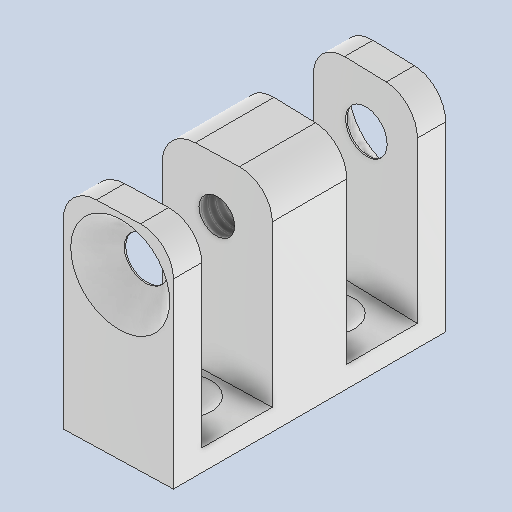
# Autodesk Inventor part: HalterUmlenkrolleDPL
Saved by Autodesk Inventor 2025 (Build 290162010, 162A)
## iProperties
Created: 2024-11-18
Part Number: HalterUmlenkrolleDPL
Material: PC/ABS-Kunststoff, 3DDruck, PLA
Document SubType Name: Modeling
Designer: Admin
Density: 1.1 g/cm^3
Appearance: Glatt - Weiß(2)
Mass: 2.69194 g
Surface Area: 21.9285 cm^2
Volume: 2.44721 cm^3
Author: Admin
Autodesk Inventor part; units mm, degrees
ref_plane "YZ Plane" through (0, 0, 0) normal (1, 0, 0) x (0, 1, 0)
ref_plane "XZ Plane" through (0, 0, 0) normal (0, 1, 0) x (-1, 0, 0)
ref_plane "XY Plane" through (0, 0, 0) normal (0, 0, 1) x (1, 0, 0)
sketch "Skizze1" plane through (0, 0, 0) normal (0, 0, 1) x (1, 0, 0)
  line L0 (12.8939, 29.9395) -> (2.8939, 30.2214)
  line L1 (2.8939, 30.2214) -> (2.8939, 27.5839)
  line L2 (2.8939, 27.5839) -> (12.8939, 27.302)
  line L3 (12.8939, 27.302) -> (12.8939, 29.9395)
  line L4 (12.8939, 7.1408) -> (2.8939, 6.8589)
  line L5 (2.8939, 6.8589) -> (2.8939, 4.2214)
  line L6 (2.8939, 4.2214) -> (12.8939, 4.5032)
  line L7 (12.8939, 4.5032) -> (12.8939, 7.1408)
  line L8 (2.8939, 20.9812) -> (12.8939, 20.6994)
  line L9 (12.8939, 13.7434) -> (2.8939, 13.4615)
  line L10 (16.8903, 10.5547) -> (7.8939, 10.3011) construction
  line L11 (16.8903, 23.888) -> (7.8939, 24.1416) construction
  line L12 (16.8903, 10.5547) -> (16.8903, 23.888) construction
  line L13 (2.8939, 20.9812) -> (12.8939, 27.302) construction
  line L14 (2.8939, 13.4615) -> (12.8939, 7.1408) construction
  line L15 (2.8939, 13.4615) -> (2.8939, 20.9812)
  line L16 (12.8939, 13.7434) -> (12.8939, 20.6994)
  point P0 (7.8939, 6.9998)
  dimension "d36" = 9
  dimension "d37" = 13.3333
  dimension "d38" = 91.615
  dimension "d39" = 91.615
  dimension "d40" = 10
  dimension "d41" = 6.6
  dimension "d42" = 6.6
  dimension "d43" = 13.8405
  dimension "d58" = 26
  constraints: 34 end point, 6 parallel, 5 collinear, 3 midpoint, 2 vertical, 1 point on line, 1 other
  measures "d36" distance of L10.end L10.start
  measures "d37" distance of L10.start L11.start
  measures "d38" angle of L12 L10
  measures "d39" angle of L12 L11
  measures "d40" distance between parallel lines of L5 L7
  measures "d41" distance between parallel lines of L9 L4
  measures "d42" distance between parallel lines of L2 L8
  measures "d43" distance of L11.end L10.end
  measures "d58" distance of L5.end L0.end
extrude "Extrusion1" add sketch "Skizze1" along normal blind 20
fillet "Rundung1" radius 3 6 edges at (12.8939, 5.822, 20) (12.8939, 28.6208, 20) (2.8939, 28.9026, 20) (2.8939, 5.5401, 20) (12.8939, 17.2214, 20) (2.8939, 17.2214, 20)
sketch "Skizze4" plane through (2.8939, 22.0416, 0) normal (0, 0, 1) x (1, 0, 0)
  line L0 (9.5, -17.8202) -> (0.5, -17.8202) construction
  line L1 (7, 7.9825) -> (3, 8.0952) construction
  line L2 (5, -11.7405) -> (5, -11.4869) construction
  line L3 (5, 1.8464) -> (5, 2.1) construction
  dimension "d59" = 13.3333
  constraints: 4 end point, 2 vertical, 1 coincident, 1 collinear
  measures "d59" distance of L2.end L3.start
sketch "Skizze6" plane through (2.8939, 4.2214, 0) normal (0, 0, -1) x (0.9992829, 0.0378646, 0)
  line L0 (10.9666, -25.3211) -> (0.9845, -25.9814) projected
  line L1 (0, 0) -> (10.0035, 0.097) projected
  line L2 (0.9845, -25.9814) -> (0, 0)
  line L3 (10.9666, -25.3211) -> (10.0035, 0.097)
  constraints: 4 end point, 1 parallel
extrude "Extrusion3" add sketch "Skizze6" against normal blind 2
hole "Bohrung4" at (7.8939, 10.5547, 0) at (7.8939, 23.888, 0) direction (0, 0, 1) diameter 2 end through all
chamfer "Fasen1" distance 1.5 angle 45 2 edges at (7.8939, 22.888, 2) (7.8939, 9.5547, 2)
sketch "Skizze7" plane through (12.8939, 4.5032, 0) normal (0.0281747, -0.999603, 0) x (0.999603, 0.0281747, 0)
  line L0 (-4.8347, 0) -> (-4.8347, 15) construction
  point P0 (-13.0156, 0)
  dimension "d60" = 15
  constraints: 2 end point, 1 coincident, 1 vertical
  measures "d60" distance of L0.start L0.end
hole "Bohrung5" at (8.0611, 4.367, 15) direction (-0.0281747, 0.999603, 0) diameter 4 depth 2.6365 countersink diameter 9 countersink angle 90
sketch "Skizze8" plane through (12.8939, 4.5032, 0) normal (0.0281747, -0.999603, 0) x (0.999603, 0.0281747, 0)
  circle A0 centre (-4.7839, 15) radius 2.0011 projected
  point P0 (-13.0156, 0)
hole "Bohrung6" at (8.1119, 4.3685, 15) direction (-0.0281747, 0.999603, 0) diameter 3.242 depth 13 tip angle 118 thread size "M4x0.7" class "6H" standard "ANSI Metric M Profile"
sketch "Skizze9" plane through (2.8939, 30.2214, 17) normal (0.0281747, 0.999603, 0) x (0.999603, -0.0281747, 0)
  line L0 (5.1693, 17) -> (5.1693, 2) construction
  point P0 (-2.0412, 17)
  dimension "d75" = 15
  constraints: 2 coincident, 2 end point, 1 vertical
  measures "d75" distance of L0.start L0.end
hole "Bohrung7" at (8.0611, 30.0757, 15) direction (-0.0281747, -0.999603, 0) diameter 4 depth 2.6365 countersink diameter 9 countersink angle 90
sketch "Skizze10" plane through (2.8939, 30.2214, 17) normal (0.0281747, 0.999603, 0) x (0.999603, -0.0281747, 0)
  circle A0 centre (5.2233, 2) radius 2.0011 projected
  point P0 (-2.0412, 17)
hole "Bohrung8" at (8.1151, 30.0742, 15) direction (-0.0281747, -0.999603, 0) diameter 3.242 depth 13 tip angle 118 thread size "M4x0.7" class "6H" standard "ANSI Metric M Profile"
